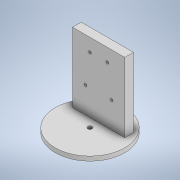
# Autodesk Inventor part: gripper
Saved by Autodesk Inventor 2022 (Build 260153000, 153)
## iProperties
Created: 2022-01-07
Part Number: gripper
Material: Generic
Document SubType Name: Modeling
Designer: nguye
Density: 1 g/cm^3
Appearance: Default
Author: nguye
Autodesk Inventor part; units mm, degrees
ref_plane "YZ Plane" through (0, 0, 0) normal (1, 0, 0) x (0, 1, 0)
ref_plane "XZ Plane" through (0, 0, 0) normal (0, 1, 0) x (-1, 0, 0)
ref_plane "XY Plane" through (0, 0, 0) normal (0, 0, 1) x (1, 0, 0)
sketch "Sketch1" plane through (0, 0, 0) normal (0, 1, 0) x (-1, 0, 0)
  circle A0 centre (0, 0) radius 40
  circle A1 centre (0, 0) radius 2.5
  dimension "d0" = 80
  dimension "d1" = 5
  constraints: 2 centre point, 2 coincident
  measures "d0" diameter of A0
  measures "d1" diameter of A1
extrude "Extrusion1" add sketch "Sketch1" along normal blind 5
sketch "Sketch2" plane through (0, 5, 0) normal (0, 1, 0) x (1, 0, 0)
  line L0 (0, 10) -> (30, 10)
  line L1 (30, 10) -> (30, 20)
  line L2 (30, 20) -> (0, 20)
  line L3 (0, 20) -> (-30, 20)
  line L4 (-30, 20) -> (-30, 10)
  line L5 (-30, 10) -> (0, 10)
  point P0 (0, 0)
  dimension "d5" = 30
  dimension "d6" = 10
  constraints: 12 end point, 2 horizontal, 2 parallel, 2 perpendicular
  measures "d5" distance of L2.end L1.end
  measures "d6" distance of L1.end L0.end
extrude "Extrusion2" add sketch "Sketch2" along normal blind 80
sketch "Sketch3" plane through (-30, 5, -10) normal (0, 0, 1) x (1, 0, 0)
  line L0 (60, 80) -> (0, 80) projected
  circle A0 centre (40, 65) radius 1.5
  circle A1 centre (20, 65) radius 1.5
  line L1 (0, 0) -> (0, 80) projected
  circle A2 centre (45, 30) radius 1.5
  circle A3 centre (15, 30) radius 1.5
  point P0 (30, -5)
  dimension "d13" = 3
  dimension "d14" = 3
  dimension "d18" = 3
  dimension "d19" = 3
  constraints: 4 centre point
  measures "d13" diameter of A0
  measures "d14" diameter of A1
  measures "d18" diameter of A2
  measures "d19" diameter of A3
extrude "Extrusion3" cut sketch "Sketch3" against normal blind 5
body "Solid1"
